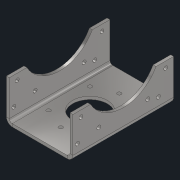
# Autodesk Inventor part: steelplate2
Saved by Autodesk Inventor 2022 (Build 260153000, 153)
## iProperties
Created: 2021-09-17
Part Number: steelplate2
Material: 鋼、炭素鋼
Document SubType Name: Sheet Metal
Designer: Yuta Kage
Density: 7.85 g/cm^3
Sheet Metal Rule: Default_mm
Appearance: 半つや出し
Author: Yuta Kage
Autodesk Inventor part; units mm, degrees
ref_plane "YZ Plane" through (0, 0, 0) normal (1, 0, 0) x (0, 1, 0)
ref_plane "XZ Plane" through (0, 0, 0) normal (0, 1, 0) x (-1, 0, 0)
ref_plane "XY Plane" through (0, 0, 0) normal (0, 0, 1) x (1, 0, 0)
sketch "スケッチ1" plane through (0, 0, 0) normal (0, 1, 0) x (-1, 0, 0)
  line L0 (30, 55) -> (-30, 55)
  line L1 (-30, 55) -> (-30, -55)
  line L2 (-30, -55) -> (30, -55)
  line L3 (30, -55) -> (30, 55)
  line L4 (30, 55) -> (-30, -55) construction
  line L5 (-30, 55) -> (30, -55) construction
  point P0 (0, 0)
  dimension "d0" = 60
  dimension "d1" = 110
  measures "d0" distance of L0.start L0.end
  measures "d1" distance of L2.end L0.start
extrude "プレート1" add sketch "スケッチ1" along normal blind 3.2
sketch "スケッチ2" plane through (-33.2, 6.4, 55) normal (-1, 0, 0) x (0, -1, 0)
  line L0 (0, -110) -> (0, 0)
  line L1 (0, 0) -> (-193.6, 0)
  line L2 (-193.6, 0) -> (-193.6, -110)
  line L3 (-193.6, -110) -> (0, -110)
  constraints: 6 end point, 1 horizontal, 1 perpendicular, 1 vertical
edge flange "フランジ1" height 200 angle 90 thickness 3.2 bend radius 3.2 thickness toward (-1, 0, 0) relief tear relief width 3.2 relief depth 1.6 corner gap 3.2 corner form 0 edges at (-30, 3.2, 0) (30, 3.2, 0) wall of the first edge with corners at (-33.2, 6.4, -55) (-33.2, 6.4, 55) (-33.2, 200, 55) (-33.2, 200, -55)
bend "曲げ1"
corner "コーナー1"
sketch "スケッチ3" plane through (36.4, 200, 55) normal (1, 0, 0) x (0, 0, -1)
  circle A0 centre (55, -135) radius 41
  line L0 (0, -200) -> (110, -200) projected
  line L1 (0, -193.6) -> (0, 0) projected
  line L2 (110, 0) -> (110, -193.6) projected
  line L3 (0, 0) -> (0, -193.6) projected
  line L4 (110, 0) -> (0, 0) projected
  line L5 (0, -155) -> (110, -155)
  line L6 (110, -155) -> (110, 0)
  line L7 (110, 0) -> (0, 0)
  line L8 (0, 0) -> (0, -155)
  point P0 (55, -200)
  point P1 (90.7911, -155)
  point P2 (110, -155)
  point P3 (0, -155)
  point P4 (19.2089, -155)
  dimension "d13" = 82
  dimension "d14" = 65
  dimension "d17" = 45
  constraints: 8 end point, 2 parallel, 1 centre point, 1 horizontal, 1 perpendicular, 1 point on line, 1 vertical alignment
  measures "d13" diameter of A0
  measures "d14" distance from line of L0 A0.centre
  measures "d17" distance between parallel lines of L0 L5
extrude "押し出し1" cut sketch "スケッチ3" against normal through all
sketch "スケッチ4" plane through (36.4, 6.4, 55) normal (1, 0, 0) x (0, 0, -1)
  arc A0 (19.2089, 38.6) -> (90.7911, 38.6) centre (55, 58.6) ccw projected
  circle A1 centre (55, 58.6) radius 53.5
  point P0 (55, -6.4)
  point P1 (55, 112.1)
  point P2 (28.25, 104.9324)
  point P3 (8.6676, 85.35)
  point P4 (1.5, 58.6)
  point P5 (8.6676, 31.85)
  point P6 (28.25, 12.2676)
  point P7 (55, 5.1)
  point P8 (81.75, 12.2676)
  point P9 (101.3324, 31.85)
  point P10 (108.5, 58.6)
  point P11 (101.3324, 85.35)
  point P12 (81.75, 104.9324)
  dimension "d18" = 107
  dimension "d21" = 360
  constraints: 2 vertical alignment, 1 coincident, 15 other
hole "穴1" at (36.4, 18.6676, 26.75) at (36.4, 38.25, 46.3324) at (36.4, 38.25, -46.3324) at (36.4, 18.6676, -26.75) direction (-1, 0, 0) diameter 4.3 end through all clearance for "Socket Head Cap Screw" size "M4" standard "Ansi Metric M Profile"
sketch "スケッチ5" plane through (36.4, 6.4, 55) normal (1, 0, 0) x (0, 0, -1)
  line L0 (0, 0) -> (0, 38.6) projected
  arc A0 (19.2089, 38.6) -> (90.7911, 38.6) centre (55, 58.6) ccw projected
  line L1 (0, 0) -> (110, 0) projected
  point P0 (55, -6.4)
  point P1 (5, 8.6)
  point P2 (93.4, 8.6)
  dimension "d30" = 88.4
  dimension "d31" = 5
  dimension "d34" = 50
  constraints: 1 horizontal alignment
  measures "d30" distance of point (5, 8.6) point (93.4, 8.6)
  measures "d31" distance from line of L0 point (5, 8.6)
  measures "d34" horizontal distance of A0.centre point (5, 8.6)
hole "穴2" at (36.4, 15, 50) at (36.4, 15, -38.4) direction (-1, 0, 0) diameter 4.3 end through all clearance for "Socket Head Cap Screw" size "M4" standard "Ansi Metric M Profile"
sketch "スケッチ6" plane through (0, 0, 0) normal (0, -1, 0) x (1, 0, 0)
  circle A0 centre (0, 0) radius 32
  point P0 (0, 32)
  point P1 (-22.6274, 22.6274)
  point P2 (-32, 0)
  point P3 (-22.6274, -22.6274)
  point P4 (0, -32)
  point P5 (22.6274, -22.6274)
  point P6 (32, 0)
  point P7 (22.6274, 22.6274)
  dimension "d42" = 64
  dimension "d45" = 360
  constraints: 1 coincident, 1 vertical alignment, 11 other
hole "穴3" at (22.6274, 0, 22.6274) at (-22.6274, 0, 22.6274) at (0, 0, 32) at (22.6274, 0, -22.6274) at (0, 0, -32) at (-22.6274, 0, -22.6274) direction (0, 1, 0) diameter 4.3 end through all clearance for "Socket Head Cap Screw" size "M4" standard "Ansi Metric M Profile"
sketch "スケッチ7" plane through (0, 3.2, 0) normal (0, 1, 0) x (1, 0, 0)
  circle A0 centre (0, 0) radius 19
  dimension "d54" = 38
  constraints: 1 centre point, 1 coincident
  measures "d54" diameter of A0
extrude "押し出し2" cut sketch "スケッチ7" against normal blind 10
equation "\"d28\" = Thickness"
equation "\"d2\" = Thickness"
equation "\"d3\" = BendReliefWidth"
equation "\"d4\" = BendReliefDepth"
equation "\"d5\" = MinimumRemnant"
equation "\"d6\" = TransitionRadius"
equation "\"d9\" = BendRadius"
equation "\"d10\" = CornerReliefSize"
equation "\"d11\" = GapSize"
equation "\"d12\" = JacobiRadiusSize"
equation "\"BendRadius\" = Thickness"
equation "\"BendReliefWidth\" = Thickness"
equation "\"BendReliefDepth\" = 0.5 * Thickness"
equation "\"CornerReliefSize\" = 4 * Thickness"
equation "\"MinimumRemnant\" = 2 * Thickness"
equation "\"TransitionRadius\" = BendRadius"
equation "\"JacobiRadiusSize\" = BendRadius"
equation "\"GapSize\" = Thickness"
equation "\"Thickness\" = 3.2"
